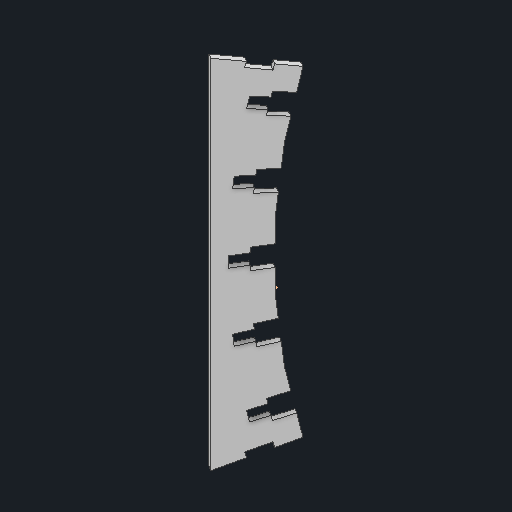
# Autodesk Inventor part: Center Plate
Saved by Autodesk Inventor 2023 (Build 270158000, 158)
## iProperties
Created: 2022-06-14
Part Number: Center Plate
Material: Generic
Document SubType Name: Modeling
Designer: FizzyApple12
Density: 1 g/cm^3
Appearance: Default
Author: FizzyApple12
Autodesk Inventor part; units mm, degrees
ref_plane "YZ Plane" through (0, 0, 0) normal (1, 0, 0) x (0, 1, 0)
ref_plane "XZ Plane" through (0, 0, 0) normal (0, 1, 0) x (-1, 0, 0)
ref_plane "XY Plane" through (0, 0, 0) normal (0, 0, 1) x (1, 0, 0)
ref_plane "Work Plane2" through (0, -19.1092, 0) normal (0.8514231, 0, 0.5244795) x (0.5130184, -0.2079117, -0.8328174)
ref_plane "Work Plane1" through (99.2081, 0, -373.4906) normal (0.8514231, 0, 0.5244795) x (0.5130184, -0.2079117, -0.8328174)
sketch "Sketch1" plane through (0, -19.1092, 0) normal (0.8514231, 0, 0.5244795) x (0.5130184, -0.2079117, -0.8328174)
  line L0 (-64.4031, -17.2568) -> (64.4031, 17.2568) construction
  line L1 (57.9081, 47.8134) -> (-73.8002, 26.9529) construction
  line L2 (-73.8887, 27.5118) -> (57.8196, 48.3724) construction
  line L3 (54.5542, 79.4406) -> (-78.6131, 72.4616) construction
  line L4 (-78.6427, 73.0267) -> (54.5245, 80.0057) construction
  line L5 (54.5245, 111.2451) -> (-78.6427, 118.2241) construction
  line L6 (64.5496, 16.7101) -> (-64.2566, -17.8034) construction
  line L7 (-50.2899, -60.7886) -> (74.2031, -13.0002) construction
  line L8 (-31.7037, -102.6067) -> (87.112, -42.0671) construction
  line L9 (74.4059, -13.5286) -> (-50.0871, -61.3169) construction
  line L10 (0.1465, -0.5466) -> (11.9566, -36.8944)
  line L11 (12.1594, -37.4227) -> (11.9566, -36.8944)
  line L12 (0, 0) -> (0.1465, -0.5466)
  line L13 (0, 0) -> (-7.946, 37.3832)
  line L14 (-8.0346, 37.9421) -> (-7.946, 37.3832)
  line L15 (12.1594, -37.4227) -> (27.7042, -72.3369)
  line L16 (-8.0346, 37.9421) -> (-12.0295, 75.9511)
  line L17 (-12.0591, 76.5162) -> (-12.0591, 114.7346)
  line L18 (-12.0591, 114.7346) -> (-51.1841, 106.4183)
  line L19 (-51.1841, 106.4183) -> (-11.4208, -80.6532)
  line L20 (-11.4208, -80.6532) -> (27.7042, -72.3369)
  line L21 (-12.0591, 76.5162) -> (-12.0295, 75.9511)
  line L22 (-5.7011, 18.3243) -> (-6.9685, 24.2871)
  line L23 (-5.7011, 18.3243) -> (-4.4336, 12.3615)
  line L24 (-6.9685, 24.2871) -> (-15.7828, 22.4135)
  line L25 (-13.2479, 10.488) -> (-4.4336, 12.3615)
  line L26 (-13.8552, 13.3451) -> (-15.1754, 19.5564) projected
  line L27 (-15.1754, 19.5564) -> (-15.7828, 22.4135)
  line L28 (-13.8552, 13.3451) -> (-13.2479, 10.488)
  line L29 (-23.1083, 11.3783) -> (-24.4286, 17.5896) projected
  line L30 (-24.4286, 17.5896) -> (-15.1754, 19.5564)
  line L31 (-13.8552, 13.3451) -> (-23.1083, 11.3783)
  line L32 (2.7351, -66.0118) -> (0.1524, -60.2107) projected
  line L33 (-12.2145, -27.9939) -> (-14.1768, -21.9547) projected
  line L34 (-29.827, 51.6736) -> (-30.4907, 57.9888) projected
  line L35 (-32.2968, 92.4504) -> (-32.2968, 98.8004) projected
  line L36 (-3.2177, -25.0707) -> (-5.1799, -19.0315) projected
  line L37 (11.3771, -62.1641) -> (8.7944, -56.3631) projected
  line L38 (-20.4189, 52.6624) -> (-21.0827, 58.9776) projected
  line L39 (-22.8369, 92.4504) -> (-22.8369, 98.8004) projected
  line L40 (2.7351, -66.0118) -> (11.3771, -62.1641)
  line L41 (8.7944, -56.3631) -> (0.1524, -60.2107)
  line L42 (-3.2177, -25.0707) -> (-12.2145, -27.9939)
  line L43 (-14.1768, -21.9547) -> (-5.1799, -19.0315)
  line L44 (-29.827, 51.6736) -> (-20.4189, 52.6624)
  line L45 (-21.0827, 58.9776) -> (-30.4907, 57.9888)
  line L46 (-32.2968, 92.4504) -> (-22.8369, 92.4504)
  line L47 (-22.8369, 98.8004) -> (-32.2968, 98.8004)
  line L48 (5.3525, -22.2861) -> (6.2551, -25.0641)
  line L49 (6.2551, -25.0641) -> (-2.315, -27.8487)
  line L50 (-2.315, -27.8487) -> (-3.2177, -25.0707)
  line L51 (3.3902, -16.2468) -> (2.4876, -13.4688)
  line L52 (2.4876, -13.4688) -> (-6.0826, -16.2534)
  line L53 (-6.0826, -16.2534) -> (-5.1799, -19.0315)
  line L54 (19.6093, -58.4989) -> (20.7973, -61.1674)
  line L55 (20.7973, -61.1674) -> (12.5652, -64.8325)
  line L56 (8.7944, -56.3631) -> (7.6063, -53.6946)
  line L57 (7.6063, -53.6946) -> (15.8384, -50.0294)
  line L58 (15.8384, -50.0294) -> (17.0265, -52.6979)
  line L59 (12.5652, -64.8325) -> (11.3771, -62.1641)
  line L60 (-11.4571, 53.6043) -> (-11.1518, 50.6993)
  line L61 (-11.1518, 50.6993) -> (-20.1136, 49.7574)
  line L62 (-20.1136, 49.7574) -> (-20.4189, 52.6624)
  line L63 (-12.1209, 59.9195) -> (-12.4262, 62.8245)
  line L64 (-12.4262, 62.8245) -> (-21.388, 61.8826)
  line L65 (-21.388, 61.8826) -> (-21.0827, 58.9776)
  line L66 (-13.8257, 92.4504) -> (-13.8257, 89.5294)
  line L67 (-13.8257, 89.5294) -> (-22.8369, 89.5294)
  line L68 (-22.8369, 89.5294) -> (-22.8369, 92.4504)
  line L69 (-22.8369, 98.8004) -> (-22.8369, 101.7214)
  line L70 (-22.8369, 101.7214) -> (-13.8257, 101.7214)
  line L71 (-13.8257, 101.7214) -> (-13.8257, 98.8004)
  line L72 (8.7177, -21.1926) -> (5.3525, -22.2861) projected
  line L73 (6.7555, -15.1534) -> (3.3902, -16.2468) projected
  line L74 (-10.2873, 92.4504) -> (-13.8257, 92.4504) projected
  line L75 (-10.2873, 98.8004) -> (-13.8257, 98.8004) projected
  line L76 (-7.938, 53.9742) -> (-11.4571, 53.6043) projected
  line L77 (-8.6018, 60.2894) -> (-12.1209, 59.9195) projected
  line L78 (22.8418, -57.0597) -> (19.6093, -58.4989) projected
  line L79 (20.259, -51.2587) -> (17.0265, -52.6979) projected
  line L80 (-13.8257, 101.7214) -> (-12.0591, 101.7214)
  line L81 (-13.8257, 89.5294) -> (-12.0591, 89.5294)
  line L82 (-12.4262, 62.8245) -> (-10.6692, 63.0092)
  line L83 (-11.1518, 50.6993) -> (-9.3948, 50.884)
  line L84 (-6.9685, 24.2871) -> (-5.2404, 24.6544)
  line L85 (-4.4336, 12.3615) -> (-2.7056, 12.7288)
  line L86 (2.4876, -13.4688) -> (4.1678, -12.9229)
  line L87 (6.2551, -25.0641) -> (7.9353, -24.5182)
  line L88 (15.8384, -50.0294) -> (17.4523, -49.3109)
  line L89 (20.7973, -61.1674) -> (22.4113, -60.4488)
  line L90 (-1.5798, 15.9543) -> (-5.041, 15.2187) projected
  line L91 (-5.041, 15.2187) -> (-6.3612, 21.4299) projected
  line L92 (-2.9001, 22.1656) -> (-6.3612, 21.4299) projected
  line L93 (-1.5798, 15.9543) -> (-2.9001, 22.1656) projected
  line L94 (-11.4571, 53.6043) -> (-12.1209, 59.9195) projected
  line L95 (-7.938, 53.9742) -> (-8.6018, 60.2894) projected
  line L96 (-13.8257, 92.4504) -> (-13.8257, 98.8004) projected
  line L97 (-10.2873, 92.4504) -> (-10.2873, 98.8004) projected
  line L98 (19.6093, -58.4989) -> (17.0265, -52.6979) projected
  line L99 (22.8418, -57.0597) -> (20.259, -51.2587) projected
  line L100 (5.3525, -22.2861) -> (3.3902, -16.2468) projected
  line L101 (8.7177, -21.1926) -> (6.7555, -15.1534) projected
  point P0 (-13.8697, 13.4133)
  point P1 (4.3713, -19.2665)
  point P2 (18.3179, -55.5984)
  point P3 (-11.789, 56.7619)
  point P4 (-13.8257, 95.6254)
  dimension "d0" = 27.94
  dimension "d16" = 6.096
  dimension "d17" = 6.096
  dimension "d20" = 6.096
  dimension "d21" = 6.096
  dimension "d22" = 6.096
  dimension "d23" = 6.096
  dimension "d24" = 6.096
  dimension "d25" = 6.096
  dimension "d26" = 6.096
  dimension "d27" = 6.096
  constraints: 124 end point, 27 perpendicular, 16 parallel, 11 midpoint, 10 point on line, 7 collinear, 1 horizontal
  measures "d0" distance between parallel lines of L19 L13
  measures "d16" distance of L22.start L22.end
  measures "d17" distance of L22.start L23.end
  measures "d20" distance from line of point (4.371, -19.266) L49
  measures "d21" distance from line of point (4.371, -19.266) L52
  measures "d22" distance from line of point (18.318, -55.598) L57
  measures "d23" distance from line of point (18.318, -55.598) L55
  measures "d24" distance from line of point (-11.789, 56.762) L61
  measures "d25" distance from line of point (-11.789, 56.762) L64
  measures "d26" distance from line of point (-13.826, 95.625) L67
  measures "d27" distance from line of point (-13.826, 95.625) L70
extrude "Extrusion1" add sketch "Sketch1" along normal blind 3.175 contours L10 L86 L52 L53 L43 L33 L42 L50 L49 L87 L11 L15 L88 L57 L56 L41 L32 L40 L59 L55 L89 L20 L19 L18 L17 L80 L70 L69 L47 L35 L46 L68 L67 L81 L21 L16 L82 L64 L65 L45 L34 L44 L62 L61 L83 L14 L13 L84 L24 L27 L30 L29 L31 L28 L25 L85 L12
sketch "Sketch3" plane through (0, -19.1092, 0) normal (-0.8514231, 0, -0.5244795) x (-0.5130184, 0.2079117, 0.8328174)
  line L0 (-5.2011, -84.1204) -> (-3.7597, -81.2915) projected
  line L1 (-16.5169, -78.3547) -> (-15.0754, -75.5258) projected
  line L2 (-26.3912, -69.7601) -> (32.4461, -99.7392) projected
  line L3 (11.4208, -80.6532) -> (-27.7042, -72.3369) projected
  line L4 (-27.7042, -72.3369) -> (-27.8194, -72.5958)
  line L5 (-27.8194, -72.5958) -> (-16.5169, -78.3547)
  line L6 (-5.2011, -84.1204) -> (9.1316, -91.4233)
  line L7 (9.1316, -91.4233) -> (11.4208, -80.6532)
  line L8 (51.1841, 106.4183) -> (11.4208, -80.6532) projected
  line L9 (-27.7042, -72.3369) -> (-12.1594, -37.4227) projected
  line L10 (37.5756, 113.1758) -> (37.4095, 116.3465) projected
  line L11 (24.893, 112.5111) -> (24.7269, 115.6818) projected
  line L12 (12.2104, 111.8465) -> (78.1546, 115.3025) projected
  line L13 (37.4095, 116.3465) -> (53.4733, 117.1883)
  line L14 (53.4733, 117.1883) -> (51.1841, 106.4183)
  line L15 (12.0591, 76.5162) -> (12.0591, 114.7346) projected
  line L16 (12.0591, 114.7346) -> (12.0591, 115.0179)
  line L17 (12.0591, 115.0179) -> (24.7269, 115.6818)
  line L18 (12.0591, 76.5162) -> (12.0591, 114.7346) projected
  line L19 (12.0591, 114.7346) -> (51.1841, 106.4183) projected
  point P0 (3.973, 18.6916)
  point P1 (-3.7597, -81.2915)
  point P2 (37.5756, 113.1758)
  point P3 (24.893, 112.5111)
  constraints: 16 end point, 4 collinear, 4 parallel
extrude "Extrusion2" add sketch "Sketch3" against normal blind 3.175
equation "\"d17\" = d16"
equation "\"d20\" = d16"
equation "\"d21\" = d16"
equation "\"d22\" = d16"
equation "\"d23\" = d16"
equation "\"d24\" = d16"
equation "\"d25\" = d16"
equation "\"d26\" = d16"
equation "\"d27\" = d16"
body "Solid1"
